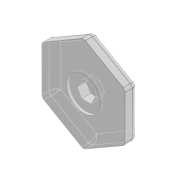
# Autodesk Inventor part: pad
Saved by Autodesk Inventor 2020 (Build 240168000, 168)
## iProperties
Created: 2020-02-17
Part Number: pad
Material: Generic
Document SubType Name: Modeling
Designer: valer
Density: 1 g/cm^3
Appearance: Default
Author: valer
Autodesk Inventor part; units mm, degrees
ref_plane "YZ Plane" through (0, 0, 0) normal (1, 0, 0) x (0, 1, 0)
ref_plane "XZ Plane" through (0, 0, 0) normal (0, 1, 0) x (-1, 0, 0)
ref_plane "XY Plane" through (0, 0, 0) normal (0, 0, 1) x (1, 0, 0)
sketch "BaseProfile" plane through (0, 0, 0) normal (0, 0, 1) x (1, 0, 0)
  circle A0 centre (0, 0) radius 4.925
  circle A1 centre (0, 0) radius 8.925
  line L0 (22.225, -12.8316) -> (0, -25.6632)
  line L1 (0, -25.6632) -> (-22.225, -12.8316)
  line L2 (-22.225, -12.8316) -> (-22.225, 12.8316)
  line L3 (-22.225, 12.8316) -> (0, 25.6632)
  line L4 (0, 25.6632) -> (22.225, 12.8316)
  line L5 (22.225, 12.8316) -> (22.225, -12.8316)
  line L6 (0, -35.9285) -> (0, 35.9285) construction
  line L7 (2.4625, 4.2652) -> (4.925, 0)
  line L8 (4.925, 0) -> (2.4625, -4.2652)
  line L9 (2.4625, -4.2652) -> (-2.4625, -4.2652)
  line L10 (-2.4625, -4.2652) -> (-4.925, 0)
  line L11 (-4.925, 0) -> (-2.4625, 4.2652)
  line L12 (-2.4625, 4.2652) -> (2.4625, 4.2652)
  dimension "d0" = 9.85
  dimension "d1" = 17.85
  dimension "d2" = 44.45
  constraints: 24 end point, 5 coincident, 1 centre point, 1 point on line, 29 other
  measures "d1" diameter of A1
  measures "d2" distance between parallel lines of L5 L2
extrude "Extrusion1" add sketch "BaseProfile" against normal blind 7 contours L7 A0 | L8 L9 L10 L11 L12 L7 | A0 L8 | L12 A0 | A0 L9 | L11 A0 | A0 L10 | A1 | L0 L1 L2 L3 L4 L5
extrude "Extrusion2" cut sketch "BaseProfile" against normal blind 1.5 contours L7 A0 | L8 L9 L10 L11 L12 L7 | A0 L8 | L12 A0 | A0 L9 | L11 A0 | A0 L10 | A1
extrude "Extrusion4" cut sketch "BaseProfile" against normal blind 6.35 contours L8 L9 L10 L11 L12 L7
fillet "Fillet1" radius 3.175 6 edges at (-11.1125, -19.2474, -7) (11.1125, -19.2474, -7) (22.225, 0, -7) (-22.225, 0, -7) (-11.1125, 19.2474, -7) (11.1125, 19.2474, -7)
fillet "Fillet2" radius 2 12 edges at (21.2951, -12.2947, -6.0701) (22.225, -12.8316, -1.9125) (21.2951, 12.2947, -6.0701) (22.225, 12.8316, -1.9125) (0, -24.5894, -6.0701) (0, -25.6632, -1.9125) (-21.2951, -12.2947, -6.0701) (-22.225, -12.8316, -1.9125) (-21.2951, 12.2947, -6.0701) (-22.225, 12.8316, -1.9125) (0, 24.5894, -6.0701) (0, 25.6632, -1.9125)
body "Solid1"
